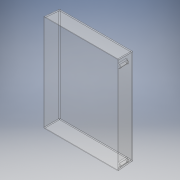
# Autodesk Inventor part: Lid
Saved by Autodesk Inventor 2017 (Build 210142000, 142)
## iProperties
Created: 2019-06-26
Part Number: Lid
Material: Polycarbonate, Clear
Document SubType Name: Modeling
Designer: Ole Simmering
Density: 1.2 g/cm^3
Appearance: Polycarbonate - Clear
Author: Ole Simmering
Autodesk Inventor part; units mm, degrees
ref_plane "YZ Plane" through (0, 0, 0) normal (1, 0, 0) x (0, 1, 0)
sketch "Sketch1" plane through (0, 0, 0) normal (0, 1, 0) x (-1, 0, 0)
  line L0 (0, 0) -> (321, 0)
  line L1 (321, 0) -> (321, -416)
  line L2 (321, -416) -> (0, -416)
  line L3 (0, -416) -> (0, 0)
  dimension "d0" = 321
  dimension "d1" = 416
  constraints: 8 end point, 2 parallel, 1 horizontal, 1 perpendicular
  measures "d0" distance of L1.end L2.end
  measures "d1" distance of L2.end L0.start
ref_plane "Work Plane1" through (0, 65, 0) normal (0, 1, 0) x (-1, 0, 0)
sketch "Sketch2" plane through (0, 65, 0) normal (0, 1, 0) x (-1, 0, 0)
  line L0 (0, 0) -> (321, 0) construction
  line L1 (321, 0) -> (321, -416) construction
  line L2 (321, -416) -> (0, -416) construction
  line L3 (0, -416) -> (0, 0) construction
  line L4 (3, -413) -> (318, -413)
  line L5 (318, -413) -> (318, -3)
  line L6 (318, -3) -> (3, -3)
  line L7 (3, -3) -> (3, -413)
  line L8 (3, -413) -> (318, -3) construction
  line L9 (318, -413) -> (3, -3) construction
  point P0 (160.5, -208)
  dimension "d3" = 315
  dimension "d4" = 410
  constraints: 12 end point, 2 midpoint, 2 parallel, 1 horizontal, 1 perpendicular
  measures "d3" distance of L6.end L5.end
  measures "d4" distance of L5.end L4.end
loft "Loft1" add profiles "Sketch1", "Sketch2"
shell "Shell1" thickness 3 removed faces 1 at (-107, 0, -277.3333)
fillet "Fillet1" radius 3 16 edges at (-1.5, 32.5, -1.5) (-3, 65, -208) (-160.5, 62, -5.8647) (-160.5, 65, -3) (-315.1353, 62, -208) (-316.566, 31, -411.566) (-160.5, 62, -410.1353) (-5.8647, 62, -208) (-160.5, 65, -413) (-318, 65, -208) (-319.5, 32.5, -414.5) (-319.5, 32.5, -1.5) (-4.434, 31, -411.566) (-1.5, 32.5, -414.5) (-4.434, 31, -4.434) (-316.566, 31, -4.434)
sketch "Sketch3" plane through (0, 0, 0) normal (0, 1, 0) x (-1, 0, 0)
  ellipse E0 centre (3.0032, -3.0032) end of major axis (0.8774, -0.8774) minor radius 3 (2.9968, 0) -> (0, -2.9968) ccw construction
  line L0 (2.9968, 0) -> (318.0032, 0) construction
  ellipse E1 centre (317.9968, -3.0032) end of major axis (320.1226, -0.8774) minor radius 3 (321, -2.9968) -> (318.0032, 0) ccw construction
  line L1 (321, -2.9968) -> (321, -413.0032) construction
  ellipse E2 centre (317.9968, -412.9968) end of major axis (320.1226, -415.1226) minor radius 3 (318.0032, -416) -> (321, -413.0032) ccw construction
  line L2 (318.0032, -416) -> (2.9968, -416) construction
  ellipse E3 centre (3.0032, -412.9968) end of major axis (0.8774, -415.1226) minor radius 3 (0, -413.0032) -> (2.9968, -416) ccw construction
  line L3 (0, -413.0032) -> (0, -2.9968) construction
  line L4 (315, -3.0032) -> (6, -3.0032) construction
  ellipse E4 centre (6.0064, -6.0064) end of major axis (3.8806, -3.8806) minor radius 3 (6, -3.0032) -> (3.0032, -6) ccw construction
  line L5 (3.0032, -6) -> (3.0032, -410) construction
  ellipse E5 centre (6.0064, -409.9936) end of major axis (3.8806, -412.1194) minor radius 3 (3.0032, -410) -> (6, -412.9968) ccw construction
  line L6 (6, -412.9968) -> (315, -412.9968) construction
  ellipse E6 centre (314.9936, -409.9936) end of major axis (317.1194, -412.1194) minor radius 3 (315, -412.9968) -> (317.9968, -410) ccw construction
  line L7 (317.9968, -410) -> (317.9968, -6) construction
  ellipse E7 centre (314.9936, -6.0064) end of major axis (317.1194, -3.8806) minor radius 3 (317.9968, -6) -> (315, -3.0032) ccw construction
  line L8 (0, -398) -> (-4, -398)
  arc A0 (-4, -384) -> (-4, -398) centre (-4, -391) ccw
  line L9 (-4, -384) -> (0, -384)
  line L10 (0, -398) -> (0, -384) construction
  line L11 (0, -398) -> (3.0032, -398)
  line L12 (3.0032, -384) -> (0, -384)
  line L13 (3.0032, -398) -> (3.0032, -384)
  point P0 (0, 0)
  dimension "d11" = 18
  dimension "d13" = 4
  dimension "d14" = 14
  constraints: 12 end point, 4 point on line, 3 perpendicular, 2 collinear, 2 point on circle, 2 tangent, 1 centre point, 1 horizontal, 8 other
  measures "d11" distance between parallel lines of L2 L8
  measures "d13" distance from line of L3 A0.centre
  measures "d14" distance between parallel lines of L9 L8
extrude "Extrusion1" add sketch "Sketch3" along normal blind 35
fillet "Fillet2" radius 4 3 edges at (-0.8077, 17.5001, -398) (-1.6154, 35, -391) (-0.8077, 17.5001, -384)
fillet "Fillet2" radius 2 3 edges at (1.1923, 35, -398) (1.1923, 35, -384) (11, 35, -391)
ref_plane "Work Plane2" through (-2.9968, 4506.6667, -208) normal (0, 0, -1) x (-1, 0, 0)
mirror "Mirror1" about plane through (-2.9968, 4506.6667, -208) normal (0, 0, -1) of "Extrusion1", "Fillet2"
sketch "Sketch4" plane through (-318.0032, 0, 0) normal (0, -1, 0) x (1, 0, 0)
  line L0 (315, -6) -> (315, -410) construction
  ellipse E0 centre (311.9968, -409.9936) end of major axis (314.1226, -412.1194) minor radius 3 (312.0032, -412.9968) -> (315, -410) ccw construction
  line L1 (312.0032, -412.9968) -> (3.0032, -412.9968) construction
  ellipse E1 centre (3.0096, -409.9936) end of major axis (0.8837, -412.1194) minor radius 3 (0.0064, -410) -> (3.0032, -412.9968) ccw construction
  line L2 (0.0064, -410) -> (0.0064, -6) construction
  ellipse E2 centre (3.0096, -6.0064) end of major axis (0.8837, -3.8806) minor radius 3 (3.0032, -3.0032) -> (0.0064, -6) ccw construction
  line L3 (3.0032, -3.0032) -> (312.0032, -3.0032) construction
  ellipse E3 centre (311.9968, -6.0064) end of major axis (314.1226, -3.8806) minor radius 3 (315, -6) -> (312.0032, -3.0032) ccw construction
  line L4 (318.0032, -14) -> (318.0032, -2.9968) construction
  ellipse E4 centre (315, -3.0032) end of major axis (317.1258, -0.8774) minor radius 3 (318.0032, -2.9968) -> (315.0064, 0) ccw construction
  line L5 (315.0064, 0) -> (0, 0) construction
  ellipse E5 centre (0.0064, -3.0032) end of major axis (-2.1195, -0.8774) minor radius 3 (0, 0) -> (-2.9968, -2.9968) ccw construction
  line L6 (-2.9968, -2.9968) -> (-2.9968, -413.0032) construction
  ellipse E6 centre (0.0064, -412.9968) end of major axis (-2.1195, -415.1226) minor radius 3 (-2.9968, -413.0032) -> (0, -416) ccw construction
  line L7 (0, -416) -> (315.0064, -416) construction
  ellipse E7 centre (315, -412.9968) end of major axis (317.1258, -415.1226) minor radius 3 (315.0064, -416) -> (318.0032, -413.0032) ccw construction
  line L8 (318.0032, -413.0032) -> (318.0032, -402) construction
  arc A0 (322.0032, -398) -> (318.0032, -402) centre (322.0032, -402) ccw construction
  arc A1 (322.0032, -398) -> (322.0032, -384) centre (322.0032, -391) ccw construction
  arc A2 (318.0032, -380) -> (322.0032, -384) centre (322.0032, -380) ccw construction
  line L9 (318.0032, -380) -> (318.0032, -36) construction
  arc A3 (322.0032, -32) -> (318.0032, -36) centre (322.0032, -36) ccw construction
  arc A4 (322.0032, -32) -> (322.0032, -18) centre (322.0032, -25) ccw construction
  arc A5 (318.0032, -14) -> (322.0032, -18) centre (322.0032, -14) ccw construction
  point P0 (318.0032, 0)
  constraints: 2 coincident, 8 other
hole "Hole1" at (4, 0, -25) at (4, 0, -391) direction (0, 1, 0) diameter 5.5 depth 30
body "Solid1"
